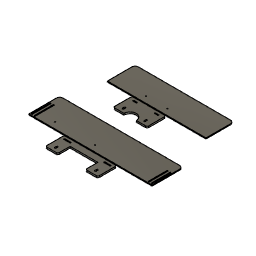
Conveyor belt walls (Autodesk Fusion 360 design; units mm, degrees)
Autodesk Fusion 360 part; units mm, degrees
sketch "Sketch3" plane through (0, 0, 0) normal (0, 0, 1) x (1, 0, 0) in component "Short wall"
  line L0 (125, -13.4) -> (115, -13.4)
  line L1 (115, -16.6) -> (125, -16.6)
  arc A0 (125, -16.6) -> (125, -13.4) centre (125, -15) ccw
  arc A1 (115, -13.4) -> (115, -16.6) centre (115, -15) ccw
  line L2 (55, -13.4) -> (45, -13.4)
  arc A2 (45, -13.4) -> (45, -16.6) centre (45, -15) ccw
  line L3 (45, -16.6) -> (55, -16.6)
  arc A3 (55, -16.6) -> (55, -13.4) centre (55, -15) ccw
  line L4 (52.1, -48.15) -> (52.1, -54.15)
  line L5 (47.9, -54.15) -> (47.9, -48.15)
  arc A4 (52.1, -48.15) -> (47.9, -48.15) centre (50, -48.15) ccw
  arc A5 (47.9, -54.15) -> (52.1, -54.15) centre (50, -54.15) ccw
  arc A6 (122.1, -48.15) -> (117.9, -48.15) centre (120, -48.15) ccw
  line L6 (122.1, -48.15) -> (122.1, -54.15)
  arc A7 (117.9, -54.15) -> (122.1, -54.15) centre (120, -54.15) ccw
  line L7 (117.9, -54.15) -> (117.9, -48.15)
  arc A8 (104.9988, -65.9318) -> (65.0012, -65.935) centre (85, -66.15) ccw
  arc A9 (140, -10) -> (135, -5) centre (135, -10) ccw
  arc A10 (135, -66.15) -> (140, -61.15) centre (135, -61.15) ccw
  arc A11 (30, -61.15) -> (35, -66.15) centre (35, -61.15) ccw
  arc A12 (35, -5) -> (30, -10) centre (35, -10) ccw
  line L8 (30, -61.15) -> (30, -10)
  line L9 (35, -66.15) -> (65.0012, -65.935)
  line L10 (35, -5) -> (135, -5)
  line L11 (140, -61.15) -> (140, -10)
  line L12 (135, -66.15) -> (104.9988, -65.9318)
  dimension "d9" = 10
  dimension "d10" = 3.2
  dimension "d11" = 10
  dimension "d12" = 3.2
  dimension "d21" = 20
  constraint horizontal L1
  constraint horizontal L3
  constraint tangent A11 L8
  constraint tangent A9 L10
  constraint tangent A10 L11
  measures "d9" distance of L0.start L0.end
  measures "d10" distance of L0.start L1.end
  measures "d11" distance of L2.end L2.start
  measures "d12" distance of L3.end L2.start
  measures "d21" radius of A8
sketch "Sketch1" plane through (0, 0, 0) normal (0, 0, 1) x (1, 0, 0) in component "Short wall"
  circle A0 centre (50, 20) radius 1.6
  circle A1 centre (120, 20) radius 1.6
  line L0 (265, 0) -> (-55, 0)
  line L1 (-55, 0) -> (-55, 80)
  line L2 (-45, 90) -> (255, 90)
  line L3 (265, 80) -> (265, 0)
  arc A2 (-45, 90) -> (-55, 80) centre (-45, 80) ccw
  arc A3 (265, 80) -> (255, 90) centre (255, 80) ccw
  dimension "d3" = 3.2
  dimension "d4" = 3.2
  dimension "d69" = 320
  dimension "d70" = 10
  dimension "d71" = 10
  constraint vertical L1
  constraint horizontal L2
  constraint vertical L3
  constraint tangent L1 A2
  constraint tangent L2 A2
  constraint tangent L3 A3
  constraint tangent L2 A3
  measures "d3" diameter of A0
  measures "d4" diameter of A1
  measures "d69" distance of L0.start L0.end
  measures "d70" radius of A2
  measures "d71" radius of A3
sketch "Sketch4" plane through (0, 0, 0) normal (0, 0, 1) x (1, 0, 0) in component "Long wall"
  arc A0 (190, -236.6) -> (190, -233.4) centre (190, -235) ccw
  line L0 (177.9, -274.15) -> (177.9, -268.15)
  arc A1 (170, -233.4) -> (170, -236.6) centre (170, -235) ccw
  arc A2 (182.1, -268.15) -> (177.9, -268.15) centre (180, -268.15) ccw
  arc A3 (60, -236.6) -> (60, -233.4) centre (60, -235) ccw
  arc A4 (40, -233.4) -> (40, -236.6) centre (40, -235) ccw
  arc A5 (177.9, -274.15) -> (182.1, -274.15) centre (180, -274.15) ccw
  arc A6 (52.1, -268.15) -> (47.9, -268.15) centre (50, -268.15) ccw
  line L1 (47.9, -274.15) -> (47.9, -268.15)
  arc A7 (47.9, -274.15) -> (52.1, -274.15) centre (50, -274.15) ccw
  line L2 (160, -246.15) -> (70, -246.15)
  line L3 (170, -233.4) -> (190, -233.4)
  line L4 (190, -236.6) -> (170, -236.6)
  line L5 (40, -233.4) -> (60, -233.4)
  line L6 (60, -236.6) -> (40, -236.6)
  arc A8 (200, -230) -> (195, -225) centre (195, -230) ccw
  arc A9 (195, -286.15) -> (200, -281.15) centre (195, -281.15) ccw
  arc A10 (160, -281.15) -> (165, -286.15) centre (165, -281.15) ccw
  arc A11 (65, -286.15) -> (70, -281.15) centre (65, -281.15) ccw
  arc A12 (30, -281.15) -> (35, -286.15) centre (35, -281.15) ccw
  arc A13 (35, -225) -> (30, -230) centre (35, -230) ccw
  line L7 (30, -281.15) -> (30, -230)
  line L8 (35, -286.15) -> (65, -286.15)
  line L9 (70, -281.15) -> (70, -246.15)
  line L10 (160, -281.15) -> (160, -246.15)
  line L11 (165, -286.15) -> (195, -286.15)
  line L12 (200, -281.15) -> (200, -230)
  line L13 (195, -225) -> (35, -225)
  line L14 (182.1, -268.15) -> (182.1, -274.15)
  line L15 (52.1, -274.15) -> (52.1, -268.15)
  dimension "d23" = 3.2
  dimension "d25" = 3.2
  constraint tangent A0 L3
  constraint tangent A1 L4
  constraint tangent A3 L5
  constraint tangent A4 L6
  constraint tangent A13 L7
  constraint tangent A11 L8
  constraint tangent A11 L9
  constraint tangent A10 L10
  constraint tangent A9 L11
  constraint tangent A8 L12
  constraint tangent A13 L13
  constraint tangent A2 L14
  constraint tangent A6 L15
  measures "d23" distance of A0.start A0.end
  measures "d25" distance of A3.start A3.end
sketch "Sketch2" plane through (0, 0, 0) normal (0, 0, 1) x (1, 0, 0) in component "Long wall"
  circle A0 centre (105, -200) radius 1.6
  circle A1 centre (-25, -200) radius 1.6
  line L0 (310, -220) -> (-90, -220)
  line L1 (-90, -220) -> (-90, -130)
  line L2 (-80, -120) -> (300, -120)
  line L3 (310, -130) -> (310, -220)
  arc A2 (310, -130) -> (300, -120) centre (300, -130) ccw
  arc A3 (-80, -120) -> (-90, -130) centre (-80, -130) ccw
  line L4 (303.4, -155) -> (303.4, -215)
  arc A4 (303.4, -215) -> (306.6, -215) centre (305, -215) ccw
  line L5 (306.6, -215) -> (306.6, -155)
  arc A5 (306.6, -155) -> (303.4, -155) centre (305, -155) ccw
  line L6 (305, -155) -> (305, -215) construction
  line L7 (293.4, -155) -> (293.4, -215)
  arc A6 (293.4, -215) -> (296.6, -215) centre (295, -215) ccw
  line L8 (296.6, -215) -> (296.6, -155)
  arc A7 (296.6, -155) -> (293.4, -155) centre (295, -155) ccw
  line L9 (295, -155) -> (295, -215) construction
  line L10 (-76.6, -155) -> (-76.6, -215)
  arc A8 (-76.6, -215) -> (-73.4, -215) centre (-75, -215) ccw
  line L11 (-73.4, -215) -> (-73.4, -155)
  arc A9 (-73.4, -155) -> (-76.6, -155) centre (-75, -155) ccw
  line L12 (-75, -155) -> (-75, -215) construction
  line L13 (-86.6, -155) -> (-86.6, -215)
  arc A10 (-86.6, -215) -> (-83.4, -215) centre (-85, -215) ccw
  line L14 (-83.4, -215) -> (-83.4, -155)
  arc A11 (-83.4, -155) -> (-86.6, -155) centre (-85, -155) ccw
  line L15 (-85, -155) -> (-85, -215) construction
  point P0 (305, -185)
  point P1 (295, -185)
  point P2 (-75, -185)
  point P3 (-85, -185)
  dimension "d7" = 3.2
  dimension "d8" = 3.2
  dimension "d65" = 10
  dimension "d66" = 10
  constraint perpendicular L1 L2
  constraint perpendicular L0 L3
  constraint tangent L3 A2
  constraint tangent L2 A2
  constraint tangent L1 A3
  constraint tangent L2 A3
  constraint tangent L4 A4
  constraint tangent A4 L5
  constraint parallel L4 L5
  constraint tangent L5 A5
  constraint tangent L4 A5
  constraint midpoint L6 P0
  constraint tangent L7 A6
  constraint tangent A6 L8
  constraint parallel L7 L8
  constraint tangent L8 A7
  constraint tangent L7 A7
  constraint midpoint L9 P1
  constraint tangent L10 A8
  constraint tangent A8 L11
  constraint parallel L10 L11
  constraint tangent L11 A9
  constraint tangent L10 A9
  constraint midpoint L12 P2
  constraint tangent L13 A10
  constraint tangent A10 L14
  constraint parallel L13 L14
  constraint tangent L14 A11
  constraint tangent L13 A11
  constraint midpoint L15 P3
  measures "d7" diameter of A0
  measures "d8" diameter of A1
  measures "d65" radius of A2
  measures "d66" radius of A3
extrude "Extrude1" add sketch "Sketch2" along normal blind 3 makes body 1 in component "Long wall"
extrude "Extrude2" add sketch "Sketch4" along normal blind 5 separate body makes body 2 in component "Long wall"
extrude "Extrude1'" add sketch "Sketch1" along normal blind 3 separate body makes body 3 in component "Short wall"
extrude "Extrude2'" add sketch "Sketch3" along normal blind 5 separate body makes body 4 in component "Short wall"
component "Short wall" placed x (1, 0, 0) y (0, 1, 0) z (0, 0, 1) at (0, 0, 0)
component "Long wall" placed x (1, 0, 0) y (0, 1, 0) z (0, 0, 1) at (0, 0, 0)
